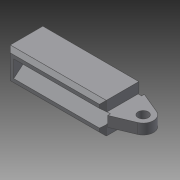
# Autodesk Inventor part: switch
Saved by Autodesk Inventor 2018 (Build 220112000, 112)
## iProperties
Created: 2019-02-20
Part Number: switch
Material: 一般
Document SubType Name: Modeling
Designer: ku_sk
Density: 1 g/cm^3
Appearance: 既定
Author: ku_sk
Autodesk Inventor part; units mm, degrees
ref_plane "YZ Plane" through (0, 0, 0) normal (1, 0, 0) x (0, 1, 0)
ref_plane "XZ Plane" through (0, 0, 0) normal (0, 1, 0) x (-1, 0, 0)
ref_plane "XY Plane" through (0, 0, 0) normal (0, 0, 1) x (1, 0, 0)
sketch "スケッチ1" plane through (0, 0, 0) normal (1, 0, 0) x (0, 1, 0)
  line L0 (5.75, 4.5) -> (-5.75, 4.5)
  line L1 (-5.75, 4.5) -> (-5.75, -4.5)
  line L2 (-5.75, -4.5) -> (5.75, -4.5)
  line L3 (5.75, -4.5) -> (5.75, 4.5)
  line L4 (-8.05, 0) -> (8.05, 0) projected
  line L5 (0, -6.3) -> (0, 6.3) projected
  point P0 (0, 0)
  point P1 (5.75, 0)
  point P2 (0, -4.5)
  dimension "d0" = 11.5
  dimension "d1" = 9
  constraints: 8 end point, 2 midpoint, 2 parallel, 2 point on line, 1 horizontal, 1 perpendicular
  measures "d0" distance of L0.start L0.end
  measures "d1" distance of L2.end L0.start
extrude "押し出し1" add sketch "スケッチ1" along normal mid plane 28
sketch "スケッチ3" plane through (0, 0, 0) normal (0, 0, 1) x (1, 0, 0)
  line L0 (14, -5.75) -> (14, 5.75) projected
  line L1 (14, -5.75) -> (21.1538, -2.7692)
  line L2 (21.1538, 2.7692) -> (14, 5.75)
  line L3 (14, 5.75) -> (14, -5.75) projected
  arc A0 (21.1538, -2.7692) -> (21.1538, 2.7692) centre (20, 0) ccw
  line L4 (-4.1, 0) -> (24.6, 0) projected
  point P0 (0, 0)
  dimension "d8" = 3
  dimension "d9" = 6
  constraints: 4 end point, 2 point on circle, 2 tangent, 1 centre point, 1 point on line
  measures "d8" radius of A0
  measures "d9" distance from line of L0 A0.centre
extrude "押し出し3" add sketch "スケッチ3" along normal blind 2.75 and the other way blind 1.75
sketch "スケッチ4" plane through (-14, 0, 0) normal (-1, 0, 0) x (0, 0, 1)
  line L0 (2.5, 5.75) -> (0, 2.75)
  line L1 (0, 2.75) -> (-2.5, 5.75)
  line L2 (-2.5, 5.75) -> (2.5, 5.75)
  line L3 (4.5, 5.75) -> (-4.5, 5.75) projected
  line L4 (0, -8.05) -> (0, 8.05) projected
  line L5 (-6.3, 0) -> (6.3, 0) projected
  line L6 (2.5, -5.75) -> (0, -2.75)
  line L7 (0, -2.75) -> (-2.5, -5.75)
  line L8 (-2.5, -5.75) -> (2.5, -5.75)
  point P0 (0, 0)
  point P1 (0, 5.75)
  point P2 (0, -5.75)
  dimension "d12" = 5
  dimension "d13" = 3
  constraints: 12 end point, 4 symmetric about line, 2 midpoint, 1 collinear, 1 horizontal, 1 point on line
  measures "d12" distance of L1.end L0.start
  measures "d13" distance from line of L2 L0.end
extrude "押し出し4" cut sketch "スケッチ4" against normal blind 29
sketch "スケッチ8" plane through (-14, 0, 0) normal (-1, 0, 0) x (0, 0, 1)
  line L0 (-6.3, 0) -> (6.3, 0) projected
  line L1 (3, 2.5) -> (1.8, 2.5)
  line L2 (1.8, 2.5) -> (1.8, -2.5)
  line L3 (1.8, -2.5) -> (3, -2.5)
  line L4 (3, -2.5) -> (3, 2.5)
  line L5 (3, 2.5) -> (1.8, -2.5) construction
  line L6 (1.8, 2.5) -> (3, -2.5) construction
  line L7 (4.5, -5.75) -> (4.5, 5.75) projected
  point P0 (0, 0)
  point P1 (2.4, 0)
  dimension "d25" = 1.2
  dimension "d26" = 1.5
  dimension "d27" = 5
  constraints: 12 end point, 2 midpoint, 2 parallel, 1 horizontal, 1 perpendicular, 1 point on line
  measures "d25" distance of L2.end L3.end
  measures "d26" distance between parallel lines of L7 L4
  measures "d27" distance of L3.end L1.start
sketch "スケッチ9" plane through (0, 0, 0) normal (0, 1, 0) x (-1, 0, 0)
  line L0 (14, 2.4) -> (0, 2.4)
  arc A0 (0, 2.4) -> (-6.9, -4.5) centre (0, -4.5) ccw
  line L1 (14, -4.5) -> (-14, -4.5) projected
  point P0 (0, 0)
  dimension "d28" = 14
  constraints: 2 end point, 2 point on circle, 1 centre point, 1 horizontal, 1 line through centre, 1 point on line, 1 tangent
  measures "d28" distance of L0.start L0.end
sweep "スイープ2" cut profiles "スケッチ8" path "スケッチ9" path curves L0 A0
sketch "スケッチ10" plane through (-14, 0, 0) normal (-1, 0, 0) x (0, 0, 1)
  line L0 (0, -8.05) -> (0, 8.05) projected
  line L1 (1.8, -2.5) -> (1.8, 2.5) projected
  line L2 (1.8, 2.5) -> (3, 2.5) projected
  line L3 (3, 2.5) -> (3, -2.5) projected
  line L4 (3, -2.5) -> (1.8, -2.5) projected
  line L5 (2.5, 5.75) -> (0, 2.75) projected
  line L6 (0, 2.75) -> (-2.5, 5.75) projected
  line L7 (-2.5, 5.75) -> (-4.5, 5.75) projected
  line L8 (-4.5, 5.75) -> (-4.5, -5.75) projected
  line L9 (-4.5, -5.75) -> (-2.5, -5.75) projected
  line L10 (-2.5, -5.75) -> (0, -2.75) projected
  line L11 (0, -2.75) -> (2.5, -5.75) projected
  line L12 (2.5, -5.75) -> (4.5, -5.75) projected
  line L13 (4.5, -5.75) -> (4.5, 5.75) projected
  line L14 (4.5, 5.75) -> (2.5, 5.75) projected
  line L15 (-1.8, -2.5) -> (-1.8, 2.5)
  line L16 (-1.8, 2.5) -> (-3, 2.5)
  line L17 (-3, 2.5) -> (-3, -2.5)
  line L18 (-3, -2.5) -> (-1.8, -2.5)
  line L19 (-1.8, 2.5) -> (-3, -2.5)
  point P0 (0, 0)
  point P1 (-2.4, 0)
  constraints: 10 end point, 4 symmetric about line, 1 midpoint
sketch "スケッチ11" plane through (0, 0, 0) normal (0, 1, 0) x (-1, 0, 0)
  line L0 (14, -2.4) -> (11, -2.4)
  arc A0 (11, -2.4) -> (8.9, -4.5) centre (11, -4.5) ccw
  line L1 (14, -4.5) -> (-14, -4.5) projected
  point P0 (0, 0)
  dimension "d31" = 3
  constraints: 2 end point, 2 point on circle, 1 centre point, 1 horizontal, 1 line through centre, 1 point on line, 1 tangent
  measures "d31" distance of L0.start L0.end
sweep "スイープ3" cut profiles "スケッチ10" path "スケッチ11" path curves L0 A0 contours L18 L19 L15 | L19 L17 L16
sketch "スケッチ12" plane through (14, 5.75, -4.5) normal (0, 0, -1) x (-1, 0, 0)
  line L0 (1.3, -3.25) -> (2.5, -3.25)
  line L1 (2.5, -3.25) -> (2.5, -8.25)
  line L2 (2.5, -8.25) -> (1.3, -8.25)
  line L3 (1.3, -8.25) -> (1.3, -3.25)
  line L4 (1.3, -3.25) -> (2.5, -8.25) construction
  line L5 (2.5, -3.25) -> (1.3, -8.25) construction
  line L6 (6.5, -3.25) -> (7.7, -3.25) projected
  line L7 (7.7, -8.25) -> (6.5, -8.25) projected
  line L8 (6.5, -8.25) -> (6.5, -3.25) projected
  line L9 (17.1, -3.25) -> (18.3, -3.25)
  line L10 (18.3, -3.25) -> (18.3, -8.25)
  line L11 (18.3, -8.25) -> (17.1, -8.25)
  line L12 (17.1, -8.25) -> (17.1, -3.25)
  line L13 (17.1, -3.25) -> (18.3, -8.25) construction
  line L14 (18.3, -3.25) -> (17.1, -8.25) construction
  line L15 (22.3, -8.25) -> (22.3, -3.25) projected
  line L16 (22.3, -3.25) -> (23.5, -3.25) projected
  line L17 (23.5, -8.25) -> (22.3, -8.25) projected
  point P0 (14, -5.75)
  point P1 (1.9, -5.75)
  point P2 (17.7, -5.75)
  dimension "d34" = 1.2
  dimension "d35" = 4
  dimension "d36" = 4
  dimension "d37" = 1.2
  constraints: 24 end point, 4 collinear, 4 midpoint, 4 parallel, 2 horizontal, 2 perpendicular
  measures "d34" distance of L0.start L0.end
  measures "d35" distance between parallel lines of L8 L1
  measures "d36" distance between parallel lines of L15 L10
  measures "d37" distance of L9.start L9.end
extrude "押し出し5" cut sketch "スケッチ12" against normal blind 4
sketch "スケッチ13" plane through (-14, 0, 0) normal (-1, 0, 0) x (0, 0, 1)
  line L0 (3, 2.5) -> (3, -2.5) projected
  line L1 (1.8, 2.5) -> (3, 2.5) projected
  line L2 (1.8, -2.5) -> (1.8, 2.5) projected
  line L3 (3, -2.5) -> (1.8, -2.5) projected
  line L4 (-1.8, 2.5) -> (-1.8, -2.5) projected
  line L5 (-1.8, -2.5) -> (-3, -2.5) projected
  line L6 (-3, -2.5) -> (-3, 2.5) projected
  line L7 (-3, 2.5) -> (-1.8, 2.5) projected
  line L8 (3.5, -3) -> (3.5, 3)
  line L9 (3.5, 3) -> (1.3, 3)
  line L10 (1.3, 3) -> (1.3, -3)
  line L11 (1.3, -3) -> (3.5, -3)
  line L12 (-1.3, -3) -> (-1.3, 3)
  line L13 (-1.3, 3) -> (-3.5, 3)
  line L14 (-3.5, 3) -> (-3.5, -3)
  line L15 (-3.5, -3) -> (-1.3, -3)
  point P0 (0, 0)
  dimension "d40" = 0.5
  dimension "d41" = 0.5
  constraints: 16 end point, 6 other
  measures "d40" distance between parallel lines of L10 L2
  measures "d41" distance between parallel lines of L4 L12
extrude "押し出し6" cut sketch "スケッチ13" against normal blind 3
sketch "スケッチ14" plane through (-14, 0, 0) normal (-1, 0, 0) x (0, 0, 1)
  line L0 (1.3, 3) -> (3.5, 3) projected
  line L1 (3.5, 3) -> (3.5, -3) projected
  line L2 (3.5, -3) -> (1.3, -3) projected
  line L3 (1.3, -3) -> (1.3, 3) projected
  line L4 (-3.5, 3) -> (-1.3, 3) projected
  line L5 (-1.3, 3) -> (-1.3, -3) projected
  line L6 (-1.3, -3) -> (-3.5, -3) projected
  line L7 (-3.5, -3) -> (-3.5, 3) projected
  line L8 (0, 2.75) -> (-2.5, 5.75) projected
  line L9 (-2.5, 5.75) -> (-4.5, 5.75) projected
  line L10 (-4.5, 5.75) -> (-4.5, -5.75) projected
  line L11 (-4.5, -5.75) -> (-2.5, -5.75) projected
  line L12 (-2.5, -5.75) -> (0, -2.75) projected
  line L13 (0, -2.75) -> (2.5, -5.75) projected
  line L14 (2.5, -5.75) -> (4.5, -5.75) projected
  line L15 (4.5, -5.75) -> (4.5, 5.75) projected
  line L16 (4.5, 5.75) -> (2.5, 5.75) projected
  line L17 (2.5, 5.75) -> (0, 2.75) projected
  line L18 (2.25, 5.45) -> (2.5, 5.75) projected
  line L19 (2.5, 5.75) -> (-2.5, 5.75)
  line L20 (2.5, -5.75) -> (-2.5, -5.75)
  point P0 (0, 0)
  constraints: 4 end point, 1 horizontal, 1 parallel
extrude "押し出し7" add sketch "スケッチ14" against normal blind 2 contours L8 L19 L17 | L12 L13 L20
chamfer "面取り1" distance 0.5 angle 45 8 edges at (-11, 0, 1.3) (-11, 3, 2.4) (-11, 0, 3.5) (-11, 3, -2.4) (-11, 0, -3.5) (-11, 0, -1.3) (-11, -3, -2.4) (-11, -3, 2.4)
chamfer "面取り2" distance 1 angle 45 10 edges at (0, 5.75, 4.5) (0, -5.75, 4.5) (0, 5.75, -4.5) (0, -5.75, -4.5) (-14, -5.75, 0) (-14, 5.75, 0) (14, -5.75, 3.625) (14, -5.75, -3.5) (14, 5.75, -3.5) (14, 5.75, 3.625)
sketch "スケッチ15" plane through (0, 0, -1.75) normal (0, 0, -1) x (-1, 0, 0)
  circle A0 centre (-20, 0) radius 1.5
  arc A1 (-21.1538, 2.7692) -> (-21.1538, -2.7692) centre (-20, 0) ccw projected
  point P0 (0, 0)
  dimension "d52" = 3
  constraints: 1 centre point, 1 concentric
  measures "d52" diameter of A0
extrude "押し出し8" cut sketch "スケッチ15" against normal blind 10
equation "\"d36\" = d35"
equation "\"d37\" = d34"
equation "\"d41\" = d40"
